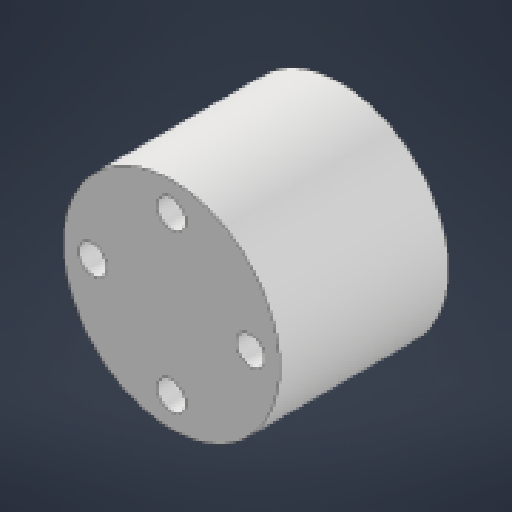
# Autodesk Inventor part: servo_rod_connector
Saved by Autodesk Inventor 2024 (Build 280153000, 153)
## iProperties
Created: 2026-03-28
Part Number: servo_rod_connector
Material: Generic
Document SubType Name: Modeling
Designer: schar
Density: 1 g/cm^3
Appearance: Default
Author: schar
Autodesk Inventor part; units mm, degrees
ref_plane "YZ Plane" through (0, 0, 0) normal (1, 0, 0) x (0, 1, 0)
ref_plane "XZ Plane" through (0, 0, 0) normal (0, 1, 0) x (-1, 0, 0)
ref_plane "XY Plane" through (0, 0, 0) normal (0, 0, 1) x (1, 0, 0)
sketch "Sketch1" plane through (0, 0, 0) normal (0, 0, 1) x (1, 0, 0)
  circle A0 centre (-10.0334, -0.6361) radius 9.6 projected
  circle A1 centre (-10.0334, 6.3639) radius 1.25 projected
  circle A2 centre (-3.0334, -0.6361) radius 1.25 projected
  circle A3 centre (-17.0334, -0.6361) radius 1.25 projected
  circle A4 centre (-10.0334, -7.6361) radius 1.25 projected
  point P0 (0, 0)
extrude "Extrusion1" add sketch "Sketch1" along normal blind 15
sketch "Sketch2" plane through (-10.0334, -0.6361, 15) normal (0, 0, 1) x (1, 0, 0)
  circle A0 centre (0, 0) radius 2.5
  point P0 (10.0334, 0.6361)
  dimension "d2" = 5
  constraints: 1 centre point
  measures "d2" diameter of A0
extrude "Extrusion2" cut sketch "Sketch2" against normal through all
ref_plane "Work Plane2" through (-10.0334, -0.6361, 15) normal (-0.866, -0.5, 0) x (0, 0, -1)
ref_plane "Work Plane1" through (54.8563, 26.4356, 21.5) normal (0.5, -0.866, 0) x (-0.2494, -0.144, -0.9577)
sketch "Sketch3" plane through (-10.0334, -0.6361, 15) normal (-0.866, -0.5, 0) x (0, 0, -1)
  line L0 (0, 9.6) -> (0, -9.6) projected
  line L1 (0, 9.6) -> (10, 9.6)
  line L2 (15, 9.6) -> (0, 9.6) projected
  line L3 (15, 9.6) -> (15, 4.6)
  line L4 (15, 9.6) -> (15, -9.6) projected
  line L5 (10, 9.6) -> (15, 4.6)
  line L6 (-3, 0) -> (18, 0) projected
  line L7 (10, 9.6) -> (0, 4.6)
  point P0 (15, 4.4658)
  point P1 (10, 9.6)
  dimension "d6" = 10
  dimension "d7" = 5
  constraints: 8 end point, 4 point on line
  measures "d6" distance of L0.start L1.end
  measures "d7" distance of L2.start L3.end
revolve "Revolution1" cut sketch "Sketch3" angle 360 about axis through (-10.0334, -0.6361, 15) along (0, 0, -1) contours L1 L7 L0
sketch "Sketch4" plane through (-10.0334, -0.6361, 0) normal (0, 0, -1) x (-1, 0, 0)
  circle A0 centre (0, 0) radius 2.5
  circle A1 centre (0, 0) radius 1.6
  point P0 (-10.0334, 0.6361)
  dimension "d9" = 3.2
  constraints: 2 centre point, 1 coincident
  measures "d9" diameter of A1
extrude "Extrusion3" add sketch "Sketch4" against normal blind 4
sketch "Sketch5" plane through (-10.0334, -0.6361, 15) normal (-0.866, -0.5, 0) x (0, 0, -1)
  line L0 (0, -2.5) -> (0, 2.5) projected
  line L1 (0, 2.5) -> (5.5, 2.5)
  line L2 (0, 2.5) -> (11, 2.5) projected
  line L3 (5.5, 2.5) -> (5.5, 8.6823)
  point P0 (15, 4.4658)
  constraints: 4 end point, 1 midpoint, 1 vertical
ref_plane "Work Plane6" through (-8.902, -1.7675, 0) normal (0.7071, -0.7071, 0) x (0, 0, -1)
ref_plane "Work Plane5" through (-10.0334, -0.6361, 15) normal (0.7071, -0.7071, 0) x (0, 0, -1)
sketch "Sketch7" plane through (-8.902, -1.7675, 0) normal (0.7071, -0.7071, 0) x (0, 0, -1)
  line L0 (-15, -2.5) -> (-15, 2.5) projected
  line L1 (-15, 0) -> (-9.5, 0)
  circle A0 centre (-9.5, 0) radius 1.5
  point P0 (0, 7.5445)
  dimension "d16" = 5.5
  dimension "d17" = 3
  constraints: 2 end point, 1 centre point, 1 coincident, 1 horizontal, 1 midpoint
  measures "d16" distance of L1.start L1.end
  measures "d17" diameter of A0
extrude "Extrusion4" cut sketch "Sketch7" along normal blind 10
sketch "Sketch8" plane through (-8.902, -1.7675, 0) normal (0.7071, -0.7071, 0) x (0, 0, -1)
  line L0 (-15, 4.6) -> (-15, -4.6) projected
  line L1 (-15, 0) -> (-9.5, 0)
  line L2 (-12.4319, 0) -> (-10.9659, 2.5391)
  line L3 (-10.9659, 2.5391) -> (-8.0341, 2.5391)
  line L4 (-8.0341, 2.5391) -> (-6.5681, 0)
  line L5 (-6.5681, 0) -> (-8.0341, -2.5391)
  line L6 (-8.0341, -2.5391) -> (-10.9659, -2.5391)
  line L7 (-10.9659, -2.5391) -> (-12.4319, 0)
  point P0 (0, 7.5445)
  point P1 (-9.6531, 1.4922)
  dimension "d20" = 5.5
  constraints: 14 end point, 1 coincident, 1 horizontal, 1 midpoint, 1 point on line, 14 other
  measures "d20" distance of L1.start L1.end
thread "Thread1" size "M3x0.5" class "6H" standard "ANSI Metric M Profile" full length
ref_plane "Work Plane4" through (-10.0334, 6.3639, 0) normal (0.7071, -0.7071, 0) x (0, 0, 1)
body "Solid1"
